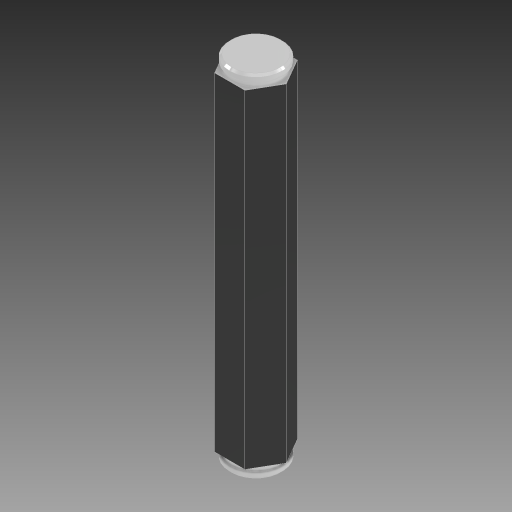
# Autodesk Inventor part: 217-2753, 3.625 in
Saved by Autodesk Inventor 2023 (Build 270158000, 158)
## iProperties
RuleStatus: InUse
AfterDocNew0: Configure
AfterModelStateActivated0: Run All
AfterAnyParamChange0: Run All
AfterAnyUserParamChange0: Run All
AfterAnyiPropertyChange0: Run All
AfterFeatureSuppressionChange0: Run All
PartBodyChanged0: Run All
Created: 2022-09-30
Material: Aluminum 7075
Document SubType Name: Modeling
Designer: Cal
Density: 2.81 g/cm^3
Appearance: Glossy - Black
Mass: 57.894 g
Surface Area: 68.1543 cm^2
Volume: 20.6028 cm^3
Author: Cal
Mass: 57.6447 g
Surface Area: 67.8749 cm^2
Volume: 20.5141 cm^3
Mass: 32.97 g
Surface Area: 40.2181 cm^2
Volume: 11.7331 cm^3
Part Number: 217-2753, 3.625 in
Autodesk Inventor part; units mm, degrees
ref_plane "YZ Plane" through (0, 0, 0) normal (1, 0, 0) x (0, 1, 0)
ref_plane "XZ Plane" through (0, 0, 0) normal (0, 1, 0) x (-1, 0, 0)
ref_plane "XY Plane" through (0, 0, 0) normal (0, 0, 1) x (1, 0, 0)
sketch "Sketch1" plane through (0, 0, 0) normal (0, 1, 0) x (-1, 0, 0)
  line L0 (-7.3323, 0) -> (-3.6662, 6.35)
  line L1 (-3.6662, 6.35) -> (3.6662, 6.35)
  line L2 (3.6662, 6.35) -> (7.3323, 0)
  line L3 (7.3323, 0) -> (3.6662, -6.35)
  line L4 (3.6662, -6.35) -> (-3.6662, -6.35)
  line L5 (-3.6662, -6.35) -> (-7.3323, 0)
  circle A0 centre (0, 0) radius 6.875
  circle A1 centre (0, 0) radius 6.35
  line L6 (-2.7496, -4.7625) -> (2.7496, -4.7625)
  line L7 (2.7496, -4.7625) -> (5.4993, 0)
  line L8 (5.4993, 0) -> (2.7496, 4.7625)
  line L9 (2.7496, 4.7625) -> (-2.7496, 4.7625)
  line L10 (-2.7496, 4.7625) -> (-5.4993, 0)
  line L11 (-5.4993, 0) -> (-2.7496, -4.7625)
  circle A2 centre (0, 0) radius 4.7625
  circle A3 centre (0, 0) radius 5.125
  circle A4 centre (0, 0) radius 9.525
  circle A5 centre (0, 0) radius 5.9436
  circle A6 centre (0, 0) radius 2.5527
  circle A7 centre (0, 0) radius 2.0193
  circle A8 centre (0, 0) radius 3.175
  circle A9 centre (0, 0) radius 8.7313
  point P0 (-4.1818, 5.457)
  point P1 (-2.635, 6.35)
  point P2 (-6.8168, -0.893)
  point P3 (-6.8168, 0.893)
  point P4 (-2.635, -6.35)
  point P5 (-4.1818, -5.457)
  point P6 (4.1818, -5.457)
  point P7 (2.635, -6.35)
  point P8 (6.8168, -0.893)
  point P9 (6.8168, 0.893)
  point P10 (2.635, 6.35)
  point P11 (4.1818, 5.457)
  point P12 (3.1778, -4.0208)
  point P13 (1.8932, -4.7625)
  point P14 (5.071, -0.7417)
  point P15 (5.071, 0.7417)
  point P16 (1.8932, 4.7625)
  point P17 (3.1778, 4.0208)
  point P18 (-3.1778, 4.0208)
  point P19 (-1.8932, 4.7625)
  point P20 (-5.071, -0.7417)
  point P21 (-5.071, 0.7417)
  point P22 (-1.8932, -4.7625)
  point P23 (-3.1778, -4.0208)
  dimension "d0" = 12.7
  dimension "d1" = 13.75
  dimension "d2" = 12.7
  dimension "d3" = 9.525
  dimension "d4" = 10.25
  dimension "d5" = 19.05
  dimension "d6" = 11.8872
  dimension "d7" = 5.1054
  dimension "d8" = 4.0386
  dimension "d9" = 6.35
  dimension "d153" = 0.7937
  constraints: 24 end point, 10 centre point, 8 coincident, 1 horizontal, 1 tangent, 18 other
  measures "d0" distance between parallel lines of L4 L1
  measures "d1" diameter of A0
  measures "d2" diameter of A1
  measures "d3" distance between parallel lines of L9 L6
  measures "d4" diameter of A3
  measures "d5" diameter of A4
  measures "d6" diameter of A5
  measures "d7" diameter of A6
  measures "d8" diameter of A7
  measures "d9" diameter of A8
  measures "d153" radial gap between concentric circles of A4 A9
extrude "BaseProfile625Round" add sketch "Sketch1" along normal mid plane 79.375 contours L0 A0 L5 | A0 L0 | L0 A1 L5 A0 | L5 A0 | L0 A0 L1 A1 | A1 | L0 L1 A0 | A1 L4 A0 L5 | A0 L4 L5 | L1 A0 | L1 A0 L2 A1 | A1 L3 A0 L4 | L4 A0 | L1 L2 A0 | L2 A0 | L2 A0 L3 A1 | A0 L3 L4 | L3 A0 | L2 L3 A0 | L11 A3 L6 | A3 L11 A2 L6 | L6 A3 | A3 L11 | A2 L7 A3 L6 | A2 | A3 L7 L6 | L11 A3 L10 A2 | L11 L10 A3 | L7 A3 | A2 L8 A3 L7 | L10 A3 | L10 A3 L9 A2 | A3 L8 L7 | L10 L9 A3 | L9 A3 | L9 A3 L8 A2 | L8 A3 | L9 L8 A3 | A4 | A5 | A6 | A7 | A8 | A9
extrude "BaseProfileRoundTube" [suppressed]
extrude "BaseProfile500Hex" cut sketch "Sketch1" against normal mid plane 914.4 contours A0 L0 | L5 A0 | L1 A0 | L4 A0 | L2 A0 | L3 A0 | A4 | A9
extrude "BaseProfile500Thunderhex" [suppressed]
extrude "BaseProfile500Round" [suppressed]
extrude "BaseProfile375Hex" [suppressed]
extrude "BaseProfile375Thunderhex" [suppressed]
extrude "BaseProfile375Round" [suppressed]
extrude "TopShaftProfile1Hex500" [suppressed]
extrude "TopShaftProfile1ThunderHex500" [suppressed]
extrude "TopShaftProfile1Round500" [suppressed]
extrude "TopShaftProfile1Hex375" [suppressed]
extrude "TopShaftProfile1ThunderHex375" [suppressed]
extrude "TopShaftProfile1Round375" [suppressed]
extrude "TopShaftProfile2ThunderHex500" [suppressed]
extrude "TopShaftProfile2Round500" [suppressed]
extrude "TopShaftProfile2Hex375" [suppressed]
extrude "TopShaftProfile2ThunderHex375" [suppressed]
extrude "TopShaftProfile2Round375" [suppressed]
sketch "Sketch2" plane through (0, 0, 0) normal (1, 0, 0) x (0, 1, 0)
  line L0 (-103.8352, 0) -> (103.8352, 0) projected
  line L1 (0, -2.6658) -> (0, 15.9951) projected
  line L2 (39.6875, 5.9436) -> (40.8305, 5.9436)
  line L3 (40.8305, 5.9436) -> (40.8305, 6.35)
  line L4 (40.8305, 6.35) -> (41.91, 6.35)
  line L5 (41.91, 6.35) -> (42.418, 5.842)
  line L6 (42.418, 5.842) -> (42.418, 0)
  line L7 (39.6875, 5.9436) -> (39.6875, 0) construction
  line L8 (39.6875, 5.9436) -> (39.6875, 6.35)
  line L9 (39.6875, 6.35) -> (39.6875, 6.35)
  line L10 (39.6875, 6.35) -> (39.6875, 0)
  line L11 (39.6875, 0) -> (42.418, 0)
  line L12 (-39.6875, 5.9436) -> (-40.8305, 5.9436)
  line L13 (-40.8305, 5.9436) -> (-40.8305, 6.35)
  line L14 (-40.8305, 6.35) -> (-41.91, 6.35)
  line L15 (-41.91, 6.35) -> (-42.418, 5.842)
  line L16 (-42.418, 5.842) -> (-42.418, 0)
  line L17 (-39.6875, 5.9436) -> (-39.6875, 0) construction
  line L18 (-39.6875, 5.9436) -> (-39.6875, 6.35)
  line L19 (-39.6875, 6.35) -> (-39.6875, 6.35)
  line L20 (-39.6875, 6.35) -> (-39.6875, 0)
  line L21 (-39.6875, 0) -> (-42.418, 0)
  line L22 (0, 0) -> (0, 13.3292)
  line L23 (39.6875, 0) -> (39.6875, 6.35)
  point P0 (-42.418, 0)
  point P1 (-39.6875, 0)
  point P2 (30.955, 4.7625)
  point P3 (-17.4625, 6.2865)
  point P4 (25.4, 4.7625)
  point P5 (19.4005, 4.7625)
  point P6 (-25.4, 4.7625)
  point P7 (-26.543, 4.7625)
  dimension "TopBearingRoundDia2" = 12.7
  dimension "d65" = 45
  dimension "RetainingRingChamferSize2" = 0.508
  dimension "d72" = 39.6875
  dimension "TopSnapRingDia2" = 11.8872
  dimension "d119" = 0.508
  dimension "d120" = 45
  dimension "d135" = 39.6875
  dimension "d138" = 42.418
  dimension "d139" = 40.8305
  dimension "d140" = 39.6875
  dimension "d141" = 11.8872
  dimension "d142" = 12.7
  dimension "d143" = 40.8305
  dimension "d144" = 39.6875
  dimension "d145" = 42.418
  constraints: 44 end point, 8 perpendicular, 5 point on line, 3 horizontal, 3 vertical, 2 collinear, 1 horizontal alignment
  measures "TopBearingRoundDia2" diameter of L4 L0
  measures "d65" angle of L4 L5
  measures "RetainingRingChamferSize2" horizontal distance of L5.end L4.end
  measures "d72" distance between parallel lines of L1 L10
  measures "TopSnapRingDia2" diameter of L2 L0
  measures "d119" horizontal distance of L15.end L14.end
  measures "d120" angle of L15 L14
  measures "d135" distance between parallel lines of L22 L20
  measures "d138" distance between parallel lines of L22 L6
  measures "d139" distance between parallel lines of L1 L3
  measures "d140" distance between parallel lines of L22 L8
  measures "d141" diameter of L12 L21
  measures "d142" diameter of L19 L0
  measures "d143" distance between parallel lines of L22 L13
  measures "d144" distance between parallel lines of L1 L18
  measures "d145" distance between parallel lines of L22 L16
revolve "TopRetentionGroove&BearingRound" add sketch "Sketch2" angle 360 about axis through (0, 0, 0) along (0, 1, 0) contours L10 L2 L3 L4 L5 L6 L0
sketch "Sketch3" plane through (0, 39.6875, 0) normal (0, 1, 0) x (1, 0, 0)
  point P0 (0, 0)
  point P1 (0, 0)
  constraints: 1 coincident
hole "TopShaftTappedHole" [suppressed]
thread "TopShaftThread" size "1/4-20 UNC" class "2B" standard "ANSI Unified Screw Threads" length 12.7
extrude "BottomShaftProfile1Hex500" [suppressed]
extrude "BottomShaftProfile1ThunderHex500" [suppressed]
extrude "BottomShaftProfile1Round500" [suppressed]
extrude "BottomShaftProfile1Hex375" [suppressed]
extrude "BottomShaftProfile1ThunderHex375" [suppressed]
extrude "BottomShaftProfile2ThunderHex500" [suppressed]
extrude "BottomShaftProfile1Round375" [suppressed]
extrude "BottomShaftProfile2Round500" [suppressed]
extrude "BottomShaftProfile2Hex375" [suppressed]
extrude "BottomShaftProfile2ThunderHex375" [suppressed]
extrude "BottomShaftProfile2Round375" [suppressed]
sketch "Sketch4" plane through (0, -39.6875, 0) normal (0, -1, 0) x (1, 0, 0)
  point P0 (0, 0)
  point P1 (0, 0)
  constraints: 1 coincident
hole "BottomShaftTappedHole" [suppressed]
thread "BottomShaftThread" size "1/4-20 UNC" class "2B" standard "ANSI Unified Screw Threads" length 12.7
revolve "BottomRetentionGroove&BearingRound" add sketch "Sketch2" angle 360 about axis through (0, -39.6875, 0) along (0, -1, 0) contours L16 L15 L14 L13 L12 L20 L0
extrude "BaseProfile375ThunderhexHole" [suppressed]
extrude "BaseProfile500ThunderhexHole" [suppressed]
equation "\"d18\" = BottomShaftProfile1Depth + TopShaftProfile1Depth + BaseShaftLength + TopShaftProfile2Depth + BottomShaftProfile2Depth"
equation "\"d72\" = 0.5 * d18"
equation "\"BaseShaftLength\" = 79.375"
equation "\"TopShaftProfile1Depth\" = 0"
equation "\"TopShaftProfile2Depth\" = 0"
equation "\"BottomShaftProfile1Depth\" = 0"
equation "\"BottomShaftProfile2Depth\" = 0"
equation "\"TopShaftHoleDia\" = 6.35"
equation "\"BottomShaftHoleDia\" = 6.35"
equation "\"TopBearingRoundDia\" = 12.7"
equation "\"TopGrooveWidth\" = 1.143"
equation "\"TopBearingRoundDistance\" = 0"
equation "\"TopSnapRingDia\" = 11.8872"
equation "\"BottomBearingRoundDia\" = 12.7"
equation "\"BottomGrooveWidth\" = 1.143"
equation "\"BottomBearingRoundDistance\" = 0"
equation "\"BottomSnapRingDia\" = 11.8872"
equation "\"RoundTubeDia\" = 19.05"
equation "\"OrderLength\" = 92.075"
body "Solid1"
body "Solid3"
